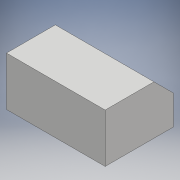
# Autodesk Inventor part: Design inkubator
Saved by Autodesk Inventor 2018 (Build 220112000, 112)
## iProperties
Created: 2018-04-17
Part Number: Design inkubator
Material: Generic
Document SubType Name: Modeling
Designer: adria
Density: 1 g/cm^3
Appearance: Default
Author: adria
Autodesk Inventor part; units mm, degrees
sketch "Sketch1" plane through (0, 0, 0) normal (0, 0, 1) x (1, 0, 0)
  line L0 (0, 0) -> (100, 0)
  line L1 (100, 0) -> (100, 50)
  line L2 (100, 50) -> (0, 50)
  line L3 (0, 50) -> (0, 0)
  dimension "d0" = 100
  dimension "d1" = 50
  constraints: 8 end point, 2 parallel, 1 horizontal, 1 perpendicular
  measures "d0" distance of L2.end L1.end
  measures "d1" distance of L1.end L0.end
sketch "Sketch2" plane through (0, 0, 0) normal (0, 1, 0) x (-1, 0, 0)
  line L0 (0, 0) -> (-100, 0)
  line L1 (-100, 0) -> (-100, -50)
  line L2 (-100, -50) -> (0, -50)
  line L3 (0, -50) -> (0, 0)
  dimension "d2" = 100
  dimension "d3" = 50
  constraints: 8 end point, 2 parallel, 1 horizontal, 1 perpendicular
  measures "d2" distance of L2.end L1.end
  measures "d3" distance of L1.end L0.end
sketch "Sketch3" plane through (0, 0, 0) normal (1, 0, 0) x (0, 1, 0)
  line L0 (0, 0) -> (50, 0)
  line L1 (50, 0) -> (50, -50)
  line L2 (50, -50) -> (0, -50)
  line L3 (0, -50) -> (0, 0)
  line L4 (50, -50) -> (70, -50)
  line L5 (70, -50) -> (70, -20)
  line L6 (70, -20) -> (50, -20)
  line L7 (70, -20) -> (50, 0)
  line L8 (70, -20) -> (69, -20)
  line L9 (50, 0) -> (50, -1)
  line L10 (50, -1) -> (69, -20)
  dimension "d16" = 50
  dimension "d17" = 50
  dimension "d18" = 20
  dimension "d19" = 30
  dimension "d20" = 1
  constraints: 22 end point, 3 parallel, 3 perpendicular, 3 point on line, 2 horizontal, 1 collinear
  measures "d16" distance of L1.end L2.end
  measures "d17" distance of L0.end L1.end
  measures "d18" distance of L1.end L4.end
  measures "d19" distance of L4.end L5.end
  measures "d20" distance of L5.end L8.end
extrude "Extrusion1" add sketch "Sketch1" against normal blind 1
extrude "Extrusion2" add sketch "Sketch2" along normal blind 1
extrude "Extrusion3" add sketch "Sketch3" along normal blind 1
ref_plane "Work Plane1" through (100, 0, 0) normal (1, 0, 0) x (0, 1, 0)
sketch "Sketch4" plane through (100, 0, 0) normal (1, 0, 0) x (0, 1, 0)
  line L0 (0, 0) -> (0, -50)
  line L1 (70, -50) -> (70, -20) projected
  line L2 (0, -50) -> (70, -50)
  line L3 (70, -50) -> (70, -20)
  line L4 (50, 0) -> (50, -1) projected
  line L5 (50, 0) -> (50, -1)
  line L6 (50, -1) -> (69, -20)
  line L7 (69, -20) -> (70, -20)
  line L8 (0, -50) -> (50, -50)
  line L9 (1, -50) -> (70, -50) projected
  line L10 (50, -1) -> (50, -50)
  line L11 (0, 0) -> (50, 0) projected
  line L12 (0, 0) -> (50, 0)
  point P0 (-1, 0)
  constraints: 18 end point, 2 parallel, 2 perpendicular, 1 collinear, 1 horizontal, 1 point on line, 1 vertical
extrude "Extrusion4" add sketch "Sketch4" along normal blind 1
ref_plane "Work Plane2" through (0, 0, -50) normal (0, 0, 1) x (1, 0, 0)
sketch "Sketch5" plane through (0, 0, -50) normal (0, 0, 1) x (1, 0, 0)
  line L0 (101, 0) -> (101, 70) projected
  line L1 (0, 0) -> (101, 0)
  line L2 (101, 0) -> (101, 70)
  line L3 (101, 70) -> (0, 70)
  line L4 (0, 70) -> (0, 0)
  dimension "d27" = 101
  dimension "d28" = 70
  constraints: 8 end point, 2 parallel, 1 horizontal, 1 perpendicular
  measures "d27" distance of L3.end L0.end
  measures "d28" distance of L0.end L1.end
sketch "Sketch6" plane through (101, 0, 0) normal (1, 0, 0) x (0, 0, -1)
  line L0 (1, 50) -> (0, 50) projected
  line L1 (20, 69) -> (1, 50) projected
  line L2 (0, 50) -> (1, 50)
  line L3 (1, 50) -> (20, 69)
  line L4 (20, 70) -> (20, 69) projected
  line L5 (20, 69) -> (20, 70)
  line L6 (20, 70) -> (0, 50)
  point P0 (0, 0)
  constraints: 8 end point, 2 collinear, 1 horizontal, 1 parallel
extrude "Extrusion5" add sketch "Sketch6" against normal blind 100
extrude "Extrusion6" add sketch "Sketch5" along normal blind 1
ref_plane "Work Plane3" through (0, 70, 0) normal (0, 1, 0) x (-1, 0, 0)
sketch "Sketch7" plane through (0, 70, 0) normal (0, 1, 0) x (-1, 0, 0)
  line L0 (0, -50) -> (-101, -50) projected
  line L1 (-101, -50) -> (-101, -20) projected
  line L2 (0, -50) -> (-101, -50)
  line L3 (-101, -50) -> (-101, -20)
  line L4 (-101, -20) -> (0, -20)
  line L5 (0, -20) -> (0, -50)
  point P0 (0, 0)
  constraints: 8 end point, 2 parallel, 1 horizontal, 1 perpendicular
extrude "Extrusion7" add sketch "Sketch7" against normal blind 1
body "Solid1"
